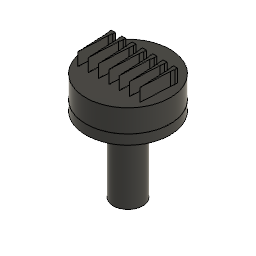
zfish-mold-D13 (Autodesk Fusion 360 design; units mm, degrees)
Autodesk Fusion 360 part; units mm, degrees
sketch "Sketch1" plane through (0, 0, 0) normal (0, 0, 1) x (1, 0, 0)
  line L0 (6.5, 3.25) -> (-6.5, 3.25) construction
  line L1 (-6.5, 3.25) -> (-6.5, -3.25) construction
  line L2 (-6.5, -3.25) -> (6.5, -3.25) construction
  line L3 (6.5, -3.25) -> (6.5, 3.25) construction
  line L4 (6.5, 3.25) -> (-6.5, -3.25) construction
  line L5 (-6.5, 3.25) -> (6.5, -3.25) construction
  line L6 (-5.1, 2.55) -> (-4.5, 2.55)
  line L7 (-4.5, 2.55) -> (-4.5, 2.15)
  line L8 (-5.1, 2.15) -> (-5.1, 2.55)
  line L9 (-4.8, 2.9409) -> (-4.8, -2.4496)
  line L10 (-5.1, 2.15) -> (-5, 1.55)
  line L11 (-4.5, 2.15) -> (-4.6, 1.55)
  line L12 (-5, 1.55) -> (-4.8, -2.95)
  line L13 (-4.6, 1.55) -> (-4.8, -2.95)
  line L14 (-3.5, 2.55) -> (-2.9, 2.55)
  line L15 (-3.5, 2.15) -> (-3.5, 2.55)
  line L16 (-3.5, 2.15) -> (-3.4, 1.55)
  line L17 (-3.4, 1.55) -> (-3.2, -2.95)
  line L18 (-3, 1.55) -> (-3.2, -2.95)
  line L19 (-2.9, 2.15) -> (-3, 1.55)
  line L20 (-2.9, 2.55) -> (-2.9, 2.15)
  line L21 (-1.9, 2.55) -> (-1.3, 2.55)
  line L22 (-1.9, 2.15) -> (-1.9, 2.55)
  line L23 (-1.9, 2.15) -> (-1.8, 1.55)
  line L24 (-1.8, 1.55) -> (-1.6, -2.95)
  line L25 (-1.4, 1.55) -> (-1.6, -2.95)
  line L26 (-1.3, 2.15) -> (-1.4, 1.55)
  line L27 (-1.3, 2.55) -> (-1.3, 2.15)
  line L28 (-0.3, 2.55) -> (0.3, 2.55)
  line L29 (-0.3, 2.15) -> (-0.3, 2.55)
  line L30 (-0.3, 2.15) -> (-0.2, 1.55)
  line L31 (-0.2, 1.55) -> (0, -2.95)
  line L32 (0.2, 1.55) -> (0, -2.95)
  line L33 (0.3, 2.15) -> (0.2, 1.55)
  line L34 (0.3, 2.55) -> (0.3, 2.15)
  line L35 (1.3, 2.55) -> (1.9, 2.55)
  line L36 (1.3, 2.15) -> (1.3, 2.55)
  line L37 (1.3, 2.15) -> (1.4, 1.55)
  line L38 (1.4, 1.55) -> (1.6, -2.95)
  line L39 (1.8, 1.55) -> (1.6, -2.95)
  line L40 (1.9, 2.15) -> (1.8, 1.55)
  line L41 (1.9, 2.55) -> (1.9, 2.15)
  line L42 (2.9, 2.55) -> (3.5, 2.55)
  line L43 (2.9, 2.15) -> (2.9, 2.55)
  line L44 (2.9, 2.15) -> (3, 1.55)
  line L45 (3, 1.55) -> (3.2, -2.95)
  line L46 (3.4, 1.55) -> (3.2, -2.95)
  line L47 (3.5, 2.15) -> (3.4, 1.55)
  line L48 (3.5, 2.55) -> (3.5, 2.15)
  line L49 (4.5, 2.55) -> (5.1, 2.55)
  line L50 (4.5, 2.15) -> (4.5, 2.55)
  line L51 (4.5, 2.15) -> (4.6, 1.55)
  line L52 (4.6, 1.55) -> (4.8, -2.95)
  line L53 (5, 1.55) -> (4.8, -2.95)
  line L54 (5.1, 2.15) -> (5, 1.55)
  line L55 (5.1, 2.55) -> (5.1, 2.15)
  circle A0 centre (0, 0) radius 6.5
  dimension "d1" = 13
  dimension "d2" = 6.5
  dimension "d3" = 0.6
  dimension "d4" = 0.4
  dimension "d5" = 0.7
  dimension "d6" = 1.4
  dimension "d7" = 0.4
  dimension "d8" = 5.5
  dimension "d9" = 0.6
  dimension "d12" = 1.6
  dimension "d13" = 0
  dimension "d20" = 13
  constraint horizontal L0
  constraint perpendicular L0 L1
  constraint parallel L0 L2
  constraint parallel L1 L3
  constraint coincident L4 A0.centre
  constraint coincident L5 A0.centre
  constraint coincident A0.centre origin
  constraint horizontal L6
  constraint vertical L7
  constraint vertical L8
  constraint perpendicular L0 L9
  constraint symmetric L7 L8 L9
  constraint horizontal L10.end L11.end
  constraint symmetric L9 L10.end L11.end
  constraint coincident L9 L12.end
  constraint equal L7 L8
  measures "d1" distance of L1.end L2.end
  measures "d2" distance of L0.end L1.end
  measures "d3" distance of L6.start L6.end
  measures "d4" distance of L6.start L8.start
  measures "d5" distance of L0 L6
  measures "d6" distance of L1 L8
  measures "d7" distance of L10.end L11.end
  measures "d8" distance of L6 L12.end
  measures "d9" vertical distance of L7.end L11.end
  measures "d20" diameter of A0
extrude "Extrude3" add sketch "Sketch1" against normal blind 5 contours L6 L7 L8 L10 L11 L12 L13 | L14 L15 L16 L17 L18 L19 L20 | L21 L22 L23 L24 L25 L26 L27 | L28 L29 L30 L31 L32 L33 L34 | L35 L36 L37 L38 L39 L40 L41 | L42 L43 L44 L45 L46 L47 L48 | L49 L50 L51 L52 L53 L54 L55 | A0 makes body 1
extrude "Extrude1" add sketch "Sketch1" along normal blind 2 contours L6 L7 L8 L10 L11 L12 L13 | L14 L15 L16 L17 L18 L19 L20 | L21 L22 L23 L24 L25 L26 L27 | L28 L29 L30 L31 L32 L33 L34 | L35 L36 L37 L38 L39 L40 L41 | L42 L43 L44 L45 L46 L47 L48 | L49 L50 L51 L52 L53 L54 L55 bodies 1
sketch "Sketch2" plane through (0, 0, -5) normal (0, 0, -1) x (1, 0, 0)
  circle A0 centre (0, 0) radius 6.5
  circle A1 centre (0, 0) radius 5
  circle A2 centre (0, 0) radius 2.3
  line L0 (-5, 0) -> (5, 0)
  line L1 (-4.1758, 2.75) -> (-1.9209, 1.265)
  line L2 (1.9209, -1.265) -> (4.1758, -2.75)
  line L3 (4.1758, 2.75) -> (1.9209, 1.265)
  line L4 (-1.9209, -1.265) -> (-4.1758, -2.75)
  arc A3 (-3.7582, 2.475) -> (-3.7582, -2.475) centre (0, 0) ccw
  arc A4 (3.7582, -2.475) -> (3.7582, 2.475) centre (0, 0) ccw
  arc A5 (-2.0879, -1.375) -> (2.0879, -1.375) centre (0, 0) ccw
  arc A6 (2.0879, 1.375) -> (-2.0879, 1.375) centre (0, 0) ccw
  line L5 (-3.9146, 2.2195) -> (-2.0692, 1.0042)
  line L6 (-3.9356, -2.1819) -> (-2.0878, -0.965)
  line L7 (2.0692, -1.0042) -> (4.333, -2.4951)
  line L8 (2.0692, 1.0042) -> (4.333, 2.4951)
  dimension "d21" = 10
  dimension "d22" = 4.6
  dimension "d23" = 5
  dimension "d24" = 5.5
  dimension "d25" = 9
  dimension "d32" = 0.3
  dimension "d33" = 0.3
  dimension "d34" = 0.3
  dimension "d35" = 0.3
  constraint concentric A0 A1
  constraint coincident A0.centre A1.centre
  constraint coincident A1 L1.start
  constraint coincident A1 L2.end
  constraint coincident A1 L3.start
  constraint coincident A1 L4.end
  constraint coincident A0.centre L3
  constraint coincident A0.centre L1
  constraint coincident A1 L0.start
  constraint coincident A1 L0.end
  constraint horizontal L0
  constraint coincident A0.centre L0
  constraint symmetric L2.end L3.start L0
  constraint concentric A1 A5
  constraint coincident A2 L1.end
  constraint collinear L1 L2
  constraint coincident A2 L4.start
  constraint collinear L3 L4
  constraint coincident A2 L2.start
  constraint coincident A2 L3.end
  constraint concentric A3 A5
  constraint coincident L3 A4.end
  constraint coincident L1 A3.start
  constraint coincident L4 A3.end
  constraint coincident L2 A4.start
  constraint concentric A3 A4
  constraint equal A3 A4
  constraint coincident L1 A6.end
  constraint coincident L4 A5.start
  constraint coincident L3 A6.start
  constraint concentric A5 A6
  constraint coincident L2 A5.end
  constraint equal A5 A6
  constraint coincident A3 L5.start
  constraint coincident A2 L5.end
  constraint coincident A3 L6.start
  constraint coincident A2 L6.end
  constraint parallel L4 L6
  constraint coincident A2 L7.start
  constraint coincident A2 L8.start
  constraint coincident A1 L8.end
  constraint coincident A1 L7.end
  constraint parallel L2 L7
  constraint parallel L3 L8
  constraint parallel L1 L5
  measures "d21" diameter of A1
  measures "d22" diameter of A2
  measures "d23" diameter of A5
  measures "d24" distance of L1.start L4.end
  measures "d25" diameter of A3
  measures "d32" distance of L1.end L5.end
  measures "d33" vertical distance of L4.start L6.end
  measures "d34" distance of L3.end L8.start
  measures "d35" distance of L2.start L7.start
extrude "Extrude4" cut sketch "Sketch2" against normal blind 3.5 contours A1 L0 A4 L8 | A1 L0 A4 L7 | A1 L3 A4 L8 | A1 L2 A4 L7 | A2 L0 A4 L7 | A2 L0 A4 L8 | A1 L1 L3 A6 | A2 L3 A4 L8 | A1 L2 L4 A5 | A2 L2 A4 L7 | A2 L0 | A2 L0 | A1 L0 L1 A3 | A1 L0 L4 A3 | A2 L0 A3 L5 | A2 L0 A3 L6 | A2 L1 A3 L5 | A2 L1 L3 A6 | A2 L4 A3 L6 | A2 L2 L4 A5 bodies 1
extrude "Extrude8" cut 1 faces at (5.9572, -0.5713, -5) along direction (0, 0, 1) blind 1.5 on bodies 1 bodies 1
extrude "Extrude5" add sketch "Sketch2" against normal blind 1.5 separate body contours A0 | A1 L1 L3 A6 | A1 L2 L4 A5 makes body 2
extrude "Extrude6" add sketch "Sketch2" along normal blind 1.4 separate body contours A2 L0 A4 L7 | A2 L0 A4 L8 | A2 L0 | A2 L0 | A2 L0 A3 L5 | A2 L0 A3 L6 makes body 3
extrude "Extrude7" add sketch "Sketch2" along normal blind 15 contours A2 L0 | A2 L0 bodies 3
fillet "Fillet1" radius 0.5 2 edges at (2.3, 0, -6.4) (-2.2999, -0.0217, -6.4) on bodies 3
fillet "Fillet2" radius 0.25 4 edges at (-2.0878, 0.965, -5.95) (2.0692, 1.0042, -5.95) (-2.0692, -1.0042, -5.95) (2.0692, -1.0042, -5.95) on bodies 3
move_body "Move1" bodies 3 to x (1, 0, 0) y (0, 1, 0) z (0, 0, 1) at (0, 0, 3.4256)
move_body "Move2" bodies 2 to x (0, 1, 0) y (-1, 0, 0) z (0, 0, 1) at (0, 0, 0)
